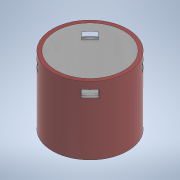
# Autodesk Inventor part: Part1
Saved by Autodesk Inventor 2022 (Build 260153000, 153)
## iProperties
Created: 2021-10-10
Part Number: Part1
Material: Generic
Document SubType Name: Modeling
Designer: Nikita
Density: 1 g/cm^3
Appearance: Default
Author: Nikita
Autodesk Inventor part; units mm, degrees
ref_plane "YZ Plane" through (0, 0, 0) normal (1, 0, 0) x (0, 1, 0)
ref_plane "XZ Plane" through (0, 0, 0) normal (0, 1, 0) x (-1, 0, 0)
sketch "Sketch1" plane through (0, 0, 0) normal (0, 1, 0) x (-1, 0, 0)
  circle A0 centre (0, 0) radius 105
  dimension "d0" = 210
  constraints: 1 centre point, 1 coincident
  measures "d0" diameter of A0
extrude "Extrusion1" add sketch "Sketch1" along normal blind 190
sketch "Sketch2" plane through (0, 190, 0) normal (0, 1, 0) x (1, 0, 0)
  circle A0 centre (0, 0) radius 95
  dimension "d3" = 190
  constraints: 1 centre point, 1 coincident
  measures "d3" diameter of A0
extrude "Extrusion2" cut sketch "Sketch2" against normal blind 170
ref_plane "Work Plane1" through (0, 170, 0) normal (0, 1, 0) x (1, 0, 0)
sketch "Sketch3" plane through (0, 170, 0) normal (0, 1, 0) x (1, 0, 0)
  circle A0 centre (0, 0) radius 95 projected
  line L0 (0, 0) -> (20.2008, 0) construction
  line L1 (0, 0) -> (20.2008, 0) construction
  circle A1 centre (0, 0) radius 105 projected
  line L2 (0, 0) -> (10.5, 0) construction
  line L3 (5.449, 7.7819) -> (60.2255, 86.011)
  line L4 (0, 0) -> (10.5, 0) construction
  line L5 (7.7819, 5.449) -> (86.011, 60.2255)
  line L6 (0, 0) -> (10.5, 0) construction
  line L7 (5.449, -7.7819) -> (60.2255, -86.011)
  line L8 (0, 0) -> (10.5, 0) construction
  line L9 (7.7819, -5.449) -> (86.011, -60.2255)
  line L10 (0, 0) -> (10.5, 0) construction
  line L11 (-5.449, 7.7819) -> (-60.2255, 86.011)
  line L12 (0, 0) -> (10.5, 0) construction
  line L13 (-7.7819, 5.449) -> (-86.011, 60.2255)
  line L14 (0, 0) -> (10.5, 0) construction
  line L15 (0, 0) -> (10.5, 0) construction
  line L16 (0, 0) -> (10.5, 0) construction
  line L17 (-5.449, -7.7819) -> (-60.2255, -86.011)
  line L18 (-7.7819, -5.449) -> (-86.011, -60.2255)
  arc A2 (7.7819, 5.449) -> (5.449, 7.7819) centre (0, 0) ccw
  arc A3 (5.449, -7.7819) -> (7.7819, -5.449) centre (0, 0) ccw
  arc A4 (-5.449, 7.7819) -> (-7.7819, 5.449) centre (0, 0) ccw
  arc A5 (-7.7819, -5.449) -> (-5.449, -7.7819) centre (0, 0) ccw
  arc A6 (-60.2255, 86.011) -> (-86.011, 60.2255) centre (0, 0) ccw
  arc A7 (86.011, 60.2255) -> (60.2255, 86.011) centre (0, 0) ccw
  arc A8 (-86.011, -60.2255) -> (-60.2255, -86.011) centre (0, 0) ccw
  arc A9 (60.2255, -86.011) -> (86.011, -60.2255) centre (0, 0) ccw
  point P0 (-77.8194, 54.4898)
  point P1 (-54.4898, 77.8194)
  point P2 (77.8194, -54.4898)
  point P3 (54.4898, -77.8194)
  point P4 (77.8194, 54.4898)
  point P5 (54.4898, 77.8194)
  point P6 (-77.8194, -54.4898)
  point P7 (-54.4898, -77.8194)
  dimension "d22" = 55
  dimension "d23" = 35
  dimension "d24" = 55
  dimension "d26" = 125
  dimension "d27" = 145
  constraints: 38 end point, 16 point on circle, 11 horizontal, 8 centre point, 3 coincident, 2 perpendicular, 9 other
  measures "d22" angle of L4 L3
  measures "d23" angle of L6 L5
  measures "d24" angle of L7 L8
  measures "d26" angle of L12 L11
  measures "d27" angle of L14 L13
extrude "Extrusion3" cut sketch "Sketch3" against normal blind 20 contours A0 L3 A1 L5 | L9 A1 L7 A0 | A0 L13 A1 L11 | L17 A1 L18 A0
body "Solid1"
